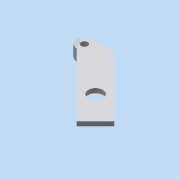
# Autodesk Inventor part: Armrechts
Saved by Autodesk Inventor 2015 (Build 190159000, 159)
## iProperties
Created: 2017-11-12
Part Number: Armrechts
Material: Generisch
Document SubType Name: Modeling
Designer: Christoph Soppa
Density: 1 g/cm^3
Appearance: Aluminium - flach
Author: Christoph Soppa
Autodesk Inventor part; units mm, degrees
ref_plane "YZ Plane" through (0, 0, 0) normal (1, 0, 0) x (0, 1, 0)
ref_plane "XZ Plane" through (0, 0, 0) normal (0, 1, 0) x (-1, 0, 0)
ref_plane "XY Plane" through (0, 0, 0) normal (0, 0, 1) x (1, 0, 0)
sketch "Skizze1" plane through (0, 0, 0) normal (0, 0, 1) x (1, 0, 0)
  arc A0 (0, 7) -> (0, -7) centre (0, 0) ccw
  line L0 (0, 7) -> (20, 7)
  line L1 (20, 7) -> (73.598, -46.598)
  line L2 (73.598, -46.598) -> (56.6274, -63.5685)
  line L3 (56.6274, -63.5685) -> (0.0589, -7)
  line L4 (0.0589, -7) -> (0, -7)
  line L5 (65.1127, -55.0833) -> (43.8995, -33.8701) construction
  circle A1 centre (43.8995, -33.8701) radius 6.5
  circle A2 centre (0, 0) radius 3.05
  dimension "d0" = 14
  dimension "d1" = 6.1
  dimension "d2" = 13
  dimension "d3" = 24
  dimension "d4" = 80
  dimension "d5" = 30
  dimension "d6" = 20
  dimension "d7" = 135
  constraints: 12 end point, 3 centre point, 3 coincident, 2 parallel, 2 perpendicular, 2 point on circle, 2 tangent, 1 horizontal, 1 midpoint
  measures "d0" diameter of A0
  measures "d1" diameter of A2
  measures "d2" diameter of A1
  measures "d3" distance of L1.end L2.end
  measures "d4" distance of L2.end L3.end
  measures "d5" distance of L5.start L5.end
  measures "d6" distance of L0.start L0.end
  measures "d7" angle of L0 L1
extrude "Extrusion1" add sketch "Skizze1" along normal blind 4
sketch "Skizze3" plane through (0, 0, 0) normal (0, 0, -1) x (-1, 0, 0)
  circle A0 centre (0, 0) radius 3.05
  circle A1 centre (0, 0) radius 7
  dimension "d14" = 14
  dimension "d15" = 6.1
  constraints: 2 centre point, 2 coincident
  measures "d14" diameter of A1
  measures "d15" diameter of A0
extrude "Extrusion3" add sketch "Skizze3" along normal blind 6
